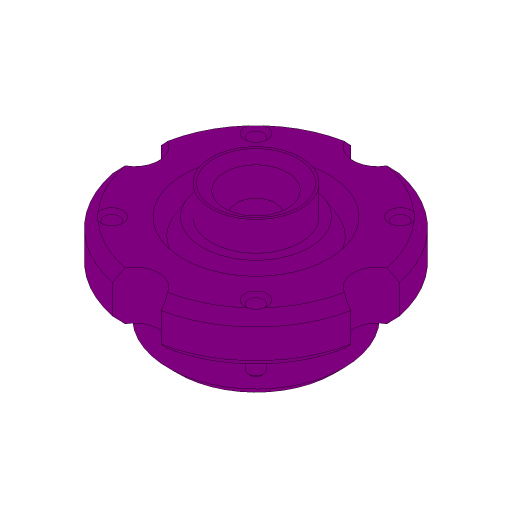
# Autodesk Inventor part: centrifugetube_adapter_20230615
Saved by Autodesk Inventor 2024 (Build 280153000, 153)
## iProperties
Created: 2022-08-29
Part Number: centrifugetube_adapter_20230615
Material: Generic
Document SubType Name: Modeling
Designer: to172
Density: 1 g/cm^3
Appearance: Smooth - Purple
Author: to172
Autodesk Inventor part; units mm, degrees
ref_plane "YZ Plane" through (0, 0, 0) normal (1, 0, 0) x (0, 1, 0)
ref_plane "XZ Plane" through (0, 0, 0) normal (0, 1, 0) x (-1, 0, 0)
ref_plane "XY Plane" through (0, 0, 0) normal (0, 0, 1) x (1, 0, 0)
sketch "Sketch1" plane through (0, 0, 0) normal (0, 0, 1) x (1, 0, 0)
  line L0 (0, 0) -> (0, 22.2922) construction
  line L1 (0, 0) -> (22.0718, 0) construction
  line L2 (2, 3.2287) -> (3.6, 6)
  line L3 (3.6, 6) -> (4.6, 6)
  line L4 (4.6, 6) -> (4.6, 3)
  line L5 (4.6, 3) -> (5.5, 3)
  line L6 (5.5, 3) -> (6.5, 1.2679)
  line L7 (6.5, 1.2679) -> (7.5, 3)
  line L8 (7.5, 3) -> (12.5, 3)
  line L9 (12.5, 3) -> (12.5, 0)
  line L10 (12.5, 0) -> (12.5, -2)
  line L11 (12.5, -2) -> (9, -2)
  line L12 (9, -2) -> (9, -7)
  line L13 (9, -7) -> (6.625, -7)
  line L14 (6.625, -7) -> (6.625, -3.5)
  line L15 (6.625, -3.5) -> (5.25, -3.5)
  line L16 (5.25, -3.5) -> (2, 0)
  line L17 (2, 3.2287) -> (2, 0)
  dimension "d0" = 12.5
  dimension "d3" = 30
  dimension "d4" = 3
  dimension "d5" = 4.6
  dimension "d6" = 1
  dimension "d7" = 6.5
  dimension "d8" = 60
  dimension "d9" = 2
  dimension "d14" = 3
  dimension "d15" = 2
  dimension "d16" = 5
  dimension "d17" = 6.625
  dimension "d18" = 9
  dimension "d19" = 2
  dimension "d21" = 3.5
  dimension "d22" = 5.25
  constraints: 36 end point, 6 perpendicular, 4 point on line, 4 vertical, 2 parallel, 1 coincident, 1 horizontal
  measures "d0" distance between parallel lines of L9 L0
  measures "d3" angle of L2 L0
  measures "d4" distance of L3.end L4.end
  measures "d5" distance between parallel lines of L4 L0
  measures "d6" distance of L2.end L3.end
  measures "d7" distance from line of L6.end L0
  measures "d8" angle of L7 L6
  measures "d9" distance of L7.end L5.end
  measures "d14" distance between parallel lines of L8 L1
  measures "d15" distance between parallel lines of L1 L11
  measures "d16" distance between parallel lines of L13 L11
  measures "d17" distance between parallel lines of L14 L0
  measures "d18" distance between parallel lines of L12 L0
  measures "d19" distance between parallel lines of L17 L0
  measures "d21" distance between parallel lines of L13 L15
  measures "d22" distance from line of L15.end L0
revolve "Revolution1" add sketch "Sketch1" angle 360 about axis through (0, 0, 0) along (0, 1, 0)
chamfer "Chamfer1" distance 0.75 angle 45 1 edges at (-3.6, 6, 0)
chamfer "Chamfer2" distance 1 angle 45 3 edges at (-12.5, 3, 0) (-12.5, -2, 0) (-9, -7, 0)
chamfer "Chamfer3" distance 0.25 angle 45 1 edges at (-6.625, -7, 0)
sketch "Sketch2" plane through (0, 3, 0) normal (0, 1, 0) x (1, 0, 0)
  circle A0 centre (0, 0) radius 10.5 construction
  line L0 (0, 0) -> (-14.6436, 0) construction
  line L1 (0, 0) -> (-11.2932, 11.2932) construction
  circle A1 centre (0, 0) radius 12.5
  circle A2 centre (-12.5, 0) radius 2.5
  circle A3 centre (-7.4246, 7.4246) radius 0.8
  point P0 (-12.25, 2.4875)
  point P1 (-12.25, -2.4875)
  point P2 (-12.25, 2.4875)
  point P3 (-12.25, -2.4875)
  dimension "d34" = 21
  dimension "d36" = 25
  dimension "d33" = 45
  dimension "d35" = 5
  dimension "d37" = 1.6
  constraints: 4 end point, 2 centre point, 2 coincident, 2 point on line, 1 horizontal, 6 other
  measures "d33" angle of L0 L1
  measures "d35" diameter of A2
  measures "d37" diameter of A3
extrude "Extrusion1" cut sketch "Sketch2" against normal blind 10 contours A2 A1 picked at (-11.6481, 0)
sketch "Sketch3" plane through (0, -2, 0) normal (0, -1, 0) x (1, 0, 0)
  circle A0 centre (0, 0) radius 10.5 construction
  line L0 (0, 0) -> (-14.6436, 0) construction
  line L1 (0, 0) -> (-11.2932, 11.2932) construction
  circle A1 centre (0, 0) radius 12.5
  circle A2 centre (-12.5, 0) radius 2.5
  circle A3 centre (-7.4246, 7.4246) radius 0.75
  point P0 (-12.25, 2.4875)
  point P1 (-12.25, -2.4875)
  point P2 (-12.25, 2.4875)
  point P3 (-12.25, -2.4875)
  dimension "d41" = 21
  dimension "d43" = 25
  dimension "d40" = 45
  dimension "d42" = 5
  dimension "d44" = 1.5
  constraints: 4 end point, 2 centre point, 2 coincident, 2 point on line, 1 horizontal, 1 horizontal alignment, 5 other
  measures "d40" angle of L0 L1
  measures "d42" diameter of A2
  measures "d44" diameter of A3
extrude "Extrusion2" cut sketch "Sketch2" against normal blind 2 contours A3
chamfer "Chamfer4" distance 0.35 angle 45 1 edges at (-8.2246, 3, -7.4246)
pattern_circular "Circular Pattern1" count 4 over 360 about axis through (0, -10, 0) along (0, 1, 0) of "Extrusion2", "Extrusion1", "Chamfer4"
extrude "Extrusion3" add sketch "Sketch3" along normal blind 1.5 contours A3
chamfer "Chamfer5" distance 0.25 angle 45 1 edges at (-8.1746, -3.5, 7.4246)
pattern_circular "Circular Pattern2" count 4 over 360 about axis through (0, -10, 0) along (0, 1, 0) of "Extrusion3", "Chamfer5"
body "Solid1"
